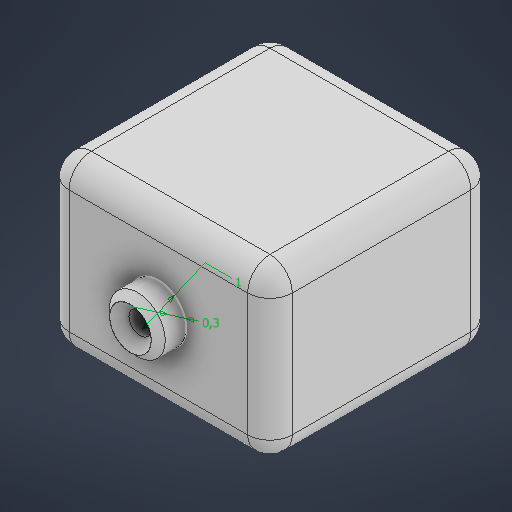
# Autodesk Inventor part: fonte IC
Saved by Autodesk Inventor 2026.2 (Build 302298010, 298A)
## iProperties
Created: 2026-03-28
Part Number: fonte IC
Material: Genérico
Document SubType Name: Modeling
Designer: Lucas David
Density: 1 g/cm^3
Appearance: Padrão
Author: Lucas David
Autodesk Inventor part; units mm, degrees
ref_plane "YZ Plane" through (0, 0, 0) normal (1, 0, 0) x (0, 1, 0)
ref_plane "XZ Plane" through (0, 0, 0) normal (0, 1, 0) x (-1, 0, 0)
ref_plane "XY Plane" through (0, 0, 0) normal (0, 0, 1) x (1, 0, 0)
sketch "Esboço1" plane through (0, 0, 0) normal (0, 0, 1) x (1, 0, 0)
  line L0 (-20, -15) -> (20, -15)
  line L1 (20, -15) -> (20, 15)
  line L2 (20, 15) -> (-20, 15)
  line L3 (-20, 15) -> (-20, -15)
  line L4 (-20, -15) -> (20, 15) construction
  line L5 (20, -15) -> (-20, 15) construction
  point P0 (0, 0)
  dimension "d0" = 30
  dimension "d1" = 40
  constraints: 12 end point, 2 midpoint, 2 parallel, 1 horizontal, 1 perpendicular
  measures "d0" distance between parallel lines of L0 L2
  measures "d1" distance between parallel lines of L1 L3
extrude "Extrusão1" add sketch "Esboço1" along normal blind 40
fillet "Arredondamento1" radius 4 12 edges at (20, 0, 40) (0, 15, 40) (0, -15, 40) (-20, 0, 40) (-20, -15, 20) (-20, 0, 0) (0, 15, 0) (-20, 15, 20) (0, -15, 0) (20, 0, 0) (20, 15, 20) (20, -15, 20)
sketch "Esboço2" plane through (0, 0, 40) normal (0, 0, 1) x (1, 0, 0)
  circle A0 centre (0, 0) radius 5
  circle A1 centre (0, 0) radius 2
  dimension "d5" = 10
  dimension "d8" = 3
  constraints: 2 centre point, 1 coincident
  measures "d5" diameter of A0
  measures "d8" radial gap between concentric circles of A0 A1
extrude "Extrusão2" add sketch "Esboço2" along normal blind 5 contours A0 | A1
extrude "Extrusão3" cut sketch "Esboço2" along normal blind 5 contours A1
chamfer "Chanfro1" distance 1.25 angle 45 1 edges at (-5, 0, 45)
chamfer "Chanfro2" distance 1.73 angle 45 1 edges at (-2, 0, 45)
